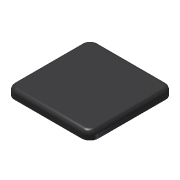
# Autodesk Inventor part: Abdeckkappe-40x40x4
Saved by Autodesk Inventor 2015 (Build 190159000, 159)
## iProperties
Created: 2016-05-04
Part Number: Abdeckkappe-40x40x4
Material: Generisch
Document SubType Name: Modeling
Designer: R. Demir
Density: 1 g/cm^3
Appearance: Dunkelgrau
Author: R. Demir
Autodesk Inventor part; units mm, degrees
ref_plane "YZ Plane" through (0, 0, 0) normal (1, 0, 0) x (0, 1, 0)
ref_plane "XZ Plane" through (0, 0, 0) normal (0, 1, 0) x (-1, 0, 0)
ref_plane "XY Plane" through (0, 0, 0) normal (0, 0, 1) x (1, 0, 0)
sketch "Skizze1" plane through (0, 0, 0) normal (0, 0, 1) x (1, 0, 0)
  line L0 (-20, 20) -> (20, 20)
  line L1 (20, 20) -> (20, -20)
  line L2 (20, -20) -> (-20, -20)
  line L3 (-20, -20) -> (-20, 20)
  line L4 (-20, 20) -> (20, -20) construction
  line L5 (20, 20) -> (-20, -20) construction
  point P0 (0, 0)
  dimension "d0" = 40
  dimension "d1" = 40
  constraints: 12 end point, 2 midpoint, 2 parallel, 1 horizontal, 1 perpendicular
  measures "d0" distance of L0.start L0.end
  measures "d1" distance of L0.end L1.end
extrude "Extrusion1" add sketch "Skizze1" along normal blind 4
fillet "Rundung1" radius 4 4 edges at (-20, -20, 2) (20, -20, 2) (-20, 20, 2) (20, 20, 2)
fillet "Rundung2" radius 2 8 edges at (18.8284, -18.8284, 4) (20, 0, 4) (18.8284, 18.8284, 4) (0, 20, 4) (-18.8284, 18.8284, 4) (-20, 0, 4) (-18.8284, -18.8284, 4) (0, -20, 4)
